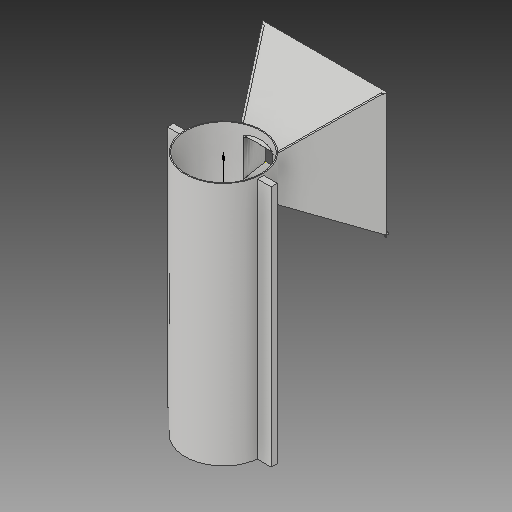
# Autodesk Inventor part: cilindro exterior
Saved by Autodesk Inventor 2019 (Build 230136000, 136)
## iProperties
Created: 2021-07-01
Part Number: cilindro exterior
Material: Genérico
Document SubType Name: Modeling
Designer: Usuario
Density: 1 g/cm^3
Appearance: Valor por defecto
Author: Usuario
Autodesk Inventor part; units mm, degrees
ref_plane "XZ Plane" through (0, 0, 0) normal (0, 1, 0) x (-1, 0, 0)
sketch "Boceto1" plane through (0, 0, 0) normal (0, 0, 1) x (1, 0, 0)
  line L0 (0, 0) -> (0, 625)
  line L1 (0, 625) -> (35, 625)
  line L2 (35, 625) -> (35, 0)
  line L3 (35, 0) -> (0, 0)
  dimension "d0" = 625
  dimension "d1" = 35
  constraints: 8 end point, 3 perpendicular, 1 vertical
  measures "d0" distance of L0.start L0.end
  measures "d1" distance of L0.end L1.end
extrude "Extrusión1" add sketch "Boceto1" along normal blind 5
sketch "Boceto2" plane through (0, 0, 0) normal (0, -1, 0) x (1, 0, 0)
  line L0 (0, 5) -> (35, 5) projected
  line L1 (35, 5) -> (133.75, 5)
  circle A0 centre (133.75, 5) radius 98.75
  line L2 (133.75, 5) -> (267.5, 5)
  line L3 (267.5, 5) -> (267.5, 0)
  line L4 (267.5, 0) -> (232.5, 0)
  line L5 (232.5, 0) -> (232.5, 5)
  circle A1 centre (133.75, 5) radius 96.25
  point P0 (0, 0)
  dimension "d5" = 197.5
  dimension "d4" = 98.75
  dimension "d6" = 133.75
  dimension "d7" = 5
  dimension "d8" = 35
  dimension "d14" = 192.5
  constraints: 10 end point, 2 coincident, 2 horizontal, 2 perpendicular, 1 centre point, 1 horizontal alignment, 1 point on line, 2 other
  measures "d4" distance of L0.end L1.end
  measures "d6" distance of L2.start L2.end
  measures "d7" distance of L2.end L3.end
  measures "d8" distance of L3.end L4.end
  measures "d14" diameter of A1
extrude "Extrusión2" add sketch "Boceto2" against normal blind 625
sketch "Boceto3" plane through (0, 0, 0) normal (0, -1, 0) x (1, 0, 0)
  arc A0 (35, 5) -> (232.5, 5) centre (133.75, 5) ccw projected
  line L0 (133.75, 5) -> (133.75, -93.75)
  circle A1 centre (133.75, 5) radius 12.5
  point P0 (0, 0)
  dimension "d11" = 25
  constraints: 2 end point, 1 centre point, 1 coincident, 1 point on circle, 1 vertical
  measures "d11" diameter of A1
extrude "Extrusión3" cut sketch "Boceto3" against normal blind 625
sketch "Boceto4" plane through (0, 625, 0) normal (0, 1, 0) x (1, 0, 0)
  circle A0 centre (133.75, -5) radius 12.5 projected
  circle A1 centre (133.75, -5) radius 96.25
  point P0 (0, 0)
  dimension "d15" = 192.5
  constraints: 1 centre point, 1 coincident
  measures "d15" diameter of A1
extrude "Extrusión4" cut sketch "Boceto4" against normal blind 620
ref_plane "Plano de trabajo1" through (133.75, 0, -93.75) normal (0, 0, 1) x (1, 0, 0)
sketch "Boceto5" plane through (133.75, 0, -93.75) normal (0, 0, 1) x (1, 0, 0)
  line L0 (98.75, 625) -> (-98.75, 625) projected
  line L1 (0, 625) -> (0, 600)
  line L2 (0, 600) -> (55, 600)
  line L3 (55, 600) -> (55, 550)
  line L4 (55, 550) -> (55, 500)
  line L5 (55, 500) -> (0, 500)
  line L6 (0, 500) -> (-55, 500)
  line L7 (-55, 500) -> (-55, 600)
  line L8 (-55, 600) -> (0, 600)
  point P0 (-133.75, 0)
  dimension "d18" = 25
  dimension "d19" = 55
  dimension "d20" = 50
  dimension "d21" = 50
  dimension "d22" = 55
  constraints: 16 end point, 5 perpendicular, 4 point on line, 1 midpoint, 1 vertical
  measures "d18" distance of L1.start L1.end
  measures "d19" distance of L1.end L2.end
  measures "d20" distance of L2.end L3.end
  measures "d21" distance of L3.end L4.end
  measures "d22" distance of L5.end L6.end
extrude "Extrusión5" cut sketch "Boceto5" along normal blind 10
ref_plane "Plano de trabajo2" through (133.75, 0, 0) normal (1, 0, 0) x (0, 1, 0)
sketch "Boceto6" plane through (133.75, 0, 0) normal (1, 0, 0) x (0, 1, 0)
  line L0 (500, -83.75) -> (600, -83.75)
  line L1 (500, -258.75) -> (218.701741, -265.847227)
  line L2 (500, -258.75) -> (941.5108, -258.75)
  line L3 (500, -83.75) -> (450.417, -169.630275)
  line L4 (500, -83.75) -> (599.166, -83.75) construction
  line L5 (450.417, -169.630275) -> (397.470182, -261.336854)
  line L6 (599.166, -83.75) -> (812.26, -83.75) construction
  line L7 (708.977475, -258.75) -> (599.166, -83.75)
  line L8 (392.471773, -261.462965) -> (495.771773, -82.542116)
  line L9 (714.880332, -258.75) -> (605.068857, -83.75)
  line L10 (500, -258.75) -> (394.038104, -258.75)
  line L11 (399.996368, -256.961371) -> (707.855121, -256.961371)
  line L12 (605.068857, -83.75) -> (600.83362, -86.407587)
  line L13 (493.540042, -86.407587) -> (497.234242, -88.540434)
  point P0 (0, 0)
  dimension "d25" = 175
  dimension "d26" = 99.166
  dimension "d27" = 120
  dimension "d30" = 206.6
  dimension "d31" = 5
  dimension "d32" = 206.6
  dimension "d33" = 5
  dimension "d34" = 1.78863
  constraints: 26 end point, 13 point on line, 3 horizontal, 3 parallel, 2 perpendicular, 1 equal length
  measures "d25" distance of L0.start L1.start
  measures "d26" distance of L0.start L3.end
  measures "d27" angle of L3 L4
  measures "d30" distance of L8.start L8.end
  measures "d31" distance of L5.end L8.start
  measures "d32" distance of L9.start L9.end
  measures "d33" distance between parallel lines of L7 L9
  measures "d34" distance between parallel lines of L11 L2
extrude "Extrusión6" add sketch "Boceto6" along normal mid plane 98 contours L3 L5 L10 L8 L13 | L12 L9 L2 L7 | L10 L5 L1 L8
sketch "Boceto9" plane through (84.75, 708.977475, -258.75) normal (0, -0.8470474, -0.5315173) x (1, 0, 0)
  line L0 (86.365969, 203.462529) -> (98, 203.462529)
  line L1 (98, 203.462529) -> (98, 0)
  line L2 (98, 203.462529) -> (98, 0)
  line L3 (98, 0) -> (0, 0)
  line L4 (98, 0) -> (0, 0)
  line L5 (98, 0) -> (209, 0)
  line L6 (0, 0) -> (-111, 0)
  line L7 (-111, 0) -> (0, 203.462529)
  line L8 (98, 203.462529) -> (209, 0)
  line L9 (0, 0) -> (0, 203.462529)
  line L10 (0, 0) -> (0, 203.462529)
  point P0 (-84.75, 596.007319)
  dimension "d40" = 111
  dimension "d41" = 111
  constraints: 14 end point, 2 collinear, 2 horizontal, 1 vertical
  measures "d40" distance of L1.end L5.end
  measures "d41" distance of L3.end L6.end
extrude "Extrusión8" add sketch "Boceto9" against normal blind 5
sketch "Boceto10" plane through (84.75, 0, 0) normal (-1, 0, 0) x (0, 0, 1)
  line L0 (-256.092413, 713.212712) -> (-258.75, 714.880332)
  line L1 (-256.092413, 713.212712) -> (-258.75, 714.880332)
  line L2 (-258.75, 714.880332) -> (-258.75, 708.977475)
  line L3 (-258.75, 708.977475) -> (-256.092413, 713.212712)
  line L4 (-258.75, 714.880332) -> (-258.75, 708.977475)
  line L5 (-258.75, 708.977475) -> (-256.092413, 713.212712)
  point P0 (0, 0)
  constraints: 7 end point, 1 collinear, 1 vertical
extrude "Extrusión9" cut sketch "Boceto10" against normal blind 300
sketch "Boceto11" plane through (84.75, 397.470182, -261.336854) normal (0, 0.8660254, -0.5) x (1, 0, 0)
  line L0 (0, 0) -> (98, 0)
  line L1 (0, 0) -> (98, 0)
  line L2 (98, 0) -> (209, 0)
  line L3 (98, 0) -> (98, -199.528119)
  line L4 (98, 0) -> (98, -199.528119)
  line L5 (98, -199.528119) -> (209, 0)
  line L6 (0, 0) -> (-111, 0)
  line L7 (0, -199.528119) -> (0, 0)
  line L8 (-111, 0) -> (0, -199.528119)
  line L9 (0, -199.528119) -> (0, 0)
  point P0 (-84.75, -27.589263)
  dimension "d46" = 98
  dimension "d47" = 111
  dimension "d48" = 111
  constraints: 14 end point, 2 horizontal, 1 collinear, 1 perpendicular, 1 point on line
  measures "d46" distance of L0.start L0.end
  measures "d47" distance of L0.end L2.end
  measures "d48" distance of L0.start L6.end
extrude "Extrusión10" add sketch "Boceto11" against normal blind 4.27
sketch "Boceto12" plane through (182.75, 0, 0) normal (1, 0, 0) x (0, 0, -1)
  line L0 (261.336854, 397.470182) -> (88.540434, 497.234242)
  line L1 (261.336854, 397.470182) -> (259.204007, 393.775983)
  line L2 (259.204007, 393.775983) -> (261.462965, 392.471773)
  line L3 (259.204007, 393.775983) -> (261.462965, 392.471773)
  line L4 (261.462965, 392.471773) -> (261.336854, 397.470182)
  line L5 (261.462965, 392.471773) -> (261.336854, 397.470182)
  point P0 (0, 0)
  constraints: 6 end point, 2 collinear, 1 perpendicular
extrude "Extrusión11" cut sketch "Boceto12" against normal blind 3000
ref_plane "Plano de trabajo6" through (0, 550, 0) normal (0, 1, 0) x (1, 0, 0)
sketch "Boceto19" plane through (0, 550, 0) normal (0, 1, 0) x (1, 0, 0)
  line L0 (-26.25, 256.092413) -> (84.75, 83.75)
  line L1 (84.75, 86.407587) -> (84.75, 83.75)
  line L2 (-26.25, 256.092413) -> (84.75, 83.75)
  line L3 (84.75, 83.75) -> (86.176529, 81.535122)
  arc A0 (232.5, -5) -> (35, -5) centre (133.75, -5) ccw
  line L4 (86.176529, 81.535122) -> (181.323471, 81.535122)
  line L5 (182.75, 83.75) -> (293.75, 256.092413)
  line L6 (181.323471, 81.535122) -> (293.75, 256.092413)
  line L7 (293.75, 256.092413) -> (-26.25, 256.092413)
  line L8 (293.75, 256.092413) -> (-26.25, 256.092413)
  line L9 (-26.25, 256.092413) -> (293.75, 256.092413)
  line L10 (92.123843, 81.535122) -> (-17.082353, 251.092413)
  line L11 (-17.082353, 251.092413) -> (284.582353, 251.092413)
  line L12 (90.44873, 83.75) -> (177.05127, 83.75)
  line L13 (86.176529, 81.535122) -> (181.323471, 81.535122)
  line L14 (182.75, 83.75) -> (90.44873, 83.75)
  line L15 (96.500839, 83.75) -> (170.999161, 83.75)
  line L16 (90.44873, 83.75) -> (-20.302686, 256.092413)
  line L17 (-26.25, 256.092413) -> (-20.302686, 256.092413)
  line L18 (287.795258, 256.092413) -> (289.502973, 258.75)
  line L19 (293.75, 258.75) -> (-26.25, 258.75)
  line L20 (171.115969, 86.407587) -> (182.75, 86.407587)
  line L21 (287.802686, 256.092413) -> (293.75, 256.092413)
  line L22 (165.400429, 88.540434) -> (182.75, 88.540434)
  line L23 (180.129511, 88.540434) -> (177.05127, 83.75)
  line L24 (284.582353, 251.092413) -> (177.05127, 83.75)
  line L25 (177.05127, 83.75) -> (284.582353, 251.092413)
  line L26 (284.582353, 251.092413) -> (287.795258, 256.092413)
  point P0 (0, 0)
  dimension "d61" = 5
  dimension "d63" = 5
  constraints: 38 end point, 8 point on line, 6 collinear, 5 horizontal, 4 point on circle
  measures "d61" distance between parallel lines of L0 L10
  measures "d63" distance between parallel lines of L7 L11
extrude "Extrusión12" add sketch "Boceto19" along normal mid plane 320 contours L7 L16 A0 L3 L0 | L7 L5 L14 L23 L24 L26 | A0 L14 L6
sketch "Boceto20" plane through (287.795258, 400.498061, -256.092413) normal (-0.8412841, 0, -0.5405933) x (-0.5405933, 0, 0.8412841)
  line L0 (0, 0) -> (0, 307.253704)
  line L1 (205.829184, 200.335559) -> (201.69742, 200.335559)
  line L2 (0, 307.253704) -> (201.69742, 200.335559)
  line L3 (205.829184, 93.041981) -> (201.69742, 93.041981)
  line L4 (201.69742, 200.335559) -> (201.69742, 93.041981)
  line L5 (0, -4.930571) -> (194.314764, 89.451138)
  line L6 (201.69742, 93.041981) -> (0, -4.930571)
  line L7 (0, -10.498061) -> (0, -4.930571)
  line L8 (0, -4.930571) -> (0, -10.498061)
  line L9 (204.856385, -10.498061) -> (0, -10.498061)
  line L10 (0, -10.498061) -> (204.856385, -10.498061)
  line L11 (204.856385, -10.498061) -> (205.829184, 93.041981)
  line L12 (2.870843, 309.501939) -> (-2.715479, 309.501939)
  line L13 (204.410203, 309.501939) -> (2.870843, 309.501939)
  line L14 (2.870843, 309.501939) -> (204.410203, 309.501939)
  line L15 (204.856385, 204.570796) -> (6.085825, 309.501939)
  line L16 (204.410203, 309.501939) -> (204.856385, 204.570796)
  line L17 (204.856385, 204.570796) -> (6.085825, 309.501939)
  point P0 (371.026655, -400.498061)
  constraints: 20 end point, 2 vertical, 1 collinear, 1 horizontal, 1 parallel, 1 perpendicular
extrude "Extrusión13" cut sketch "Boceto20" against normal blind 320
sketch "Boceto31" plane through (-20.302686, 400.498061, -256.092413) normal (0.8412676, 0, -0.540619) x (-0.540619, 0, -0.8412676)
  line L0 (-204.414072, -10.498061) -> (3.215231, -10.498061)
  line L1 (-204.8604, -10.498061) -> (-204.8604, 99.501939)
  line L2 (7.627208, -3.027879) -> (-165.370858, -3.027879)
  line L3 (2.135385, -4.930571) -> (5.831102, -6.725807)
  line L4 (7.627208, -3.027879) -> (5.831102, -6.725807)
  line L5 (0, -10.498061) -> (-204.8604, -10.498061)
  line L6 (0, -10.498061) -> (-204.414072, -10.498061)
  line L7 (-204.8604, 99.501939) -> (-208.132285, 99.501939)
  line L8 (-204.414072, -10.498061) -> (-204.8604, 99.501939)
  line L9 (-194.319279, 89.451481) -> (0, -4.930571)
  line L10 (-204.8604, 99.501939) -> (0, -4.930571)
  line L11 (0, -4.930571) -> (0, -10.498061)
  point P0 (-226.418262, -400.498061)
  constraints: 10 end point, 1 collinear
extrude "Extrusión21" cut sketch "Boceto31" against normal blind 175 contours L8 L10 L2 L9 L11 L0 | L9 L2 L10
sketch "Boceto32" plane through (90.44873, 625, -83.75) normal (0.8412676, 0, -0.540619) x (-0.540619, 0, -0.8412676)
  line L0 (0.446328, 0) -> (0.446328, 85)
  line L1 (201.985694, 85) -> (0.446328, 85)
  line L2 (0.446328, 85) -> (201.985694, 85)
  line L3 (0, -25) -> (0, -19.931143)
  line L4 (201.985694, 85) -> (0, -19.931143)
  line L5 (0, 0) -> (0, 85)
  line L6 (0, 85) -> (0, -19.931143)
  line L7 (0, 85) -> (1.071476, 85)
  point P0 (-21.557862, -625)
  constraints: 8 end point, 1 horizontal, 1 point on line
extrude "Extrusión22" cut sketch "Boceto32" against normal blind 175
sketch "Boceto33" plane through (177.05127, 605.068857, -83.75) normal (0.5405884, -0.0042521, -0.8412765) x (-0.8412841, 0, -0.5405933)
  line L0 (-4.791483, 104.932091) -> (0, 104.932091)
  line L1 (-4.791483, 104.932091) -> (0, 104.932091)
  line L2 (0, 19.930963) -> (0, 104.930194)
  line L3 (0, 104.932091) -> (0, 19.930963)
  ellipse E0 centre (-11.548986, 19.513949) end of major axis (-110.298986, 19.513949) minor radius 0.419895 (0, 19.930963) -> (-0.743957, 19.931323) ccw
  line L4 (0, 19.930963) -> (0, 19.930963)
  line L5 (0, 19.930963) -> (0, 19.930963)
  line L6 (-0.743957, 19.931323) -> (-4.791483, 104.932091)
  line L7 (0, 19.930963) -> (0, 0)
  line L8 (-0.743957, 19.931323) -> (0, 19.930963)
  point P0 (103.675725, -605.76996)
  constraints: 12 end point, 2 collinear, 2 perpendicular, 1 other
extrude "Extrusión23" cut sketch "Boceto33" against normal blind 10
sketch "Boceto35" plane through (90.207437, 390, -84.125481) normal (-0.5406145, 0.0040575, -0.8412607) x (-0.8412676, 0, 0.540619)
  ellipse E0 centre (11.551977, 0.399737) end of major axis (-87.198023, 0.399737) minor radius 0.400677 (0, 0.001811) -> (4.791469, 0) ccw
  line L0 (0, 0.001811) -> (4.791469, 0)
  line L1 (0, 0.001811) -> (0, 215.068898)
  line L2 (4.791469, 0) -> (0, 110.000905)
  line L3 (0, 110.000905) -> (0, 0.001811)
  line L4 (0, 0.001811) -> (4.791469, 0)
  point P0 (121.368422, -389.907508)
  constraints: 8 end point, 1 collinear, 1 other
extrude "Extrusión25" cut sketch "Boceto35" against normal blind 10
sketch "Boceto36" plane through (133.75, 5, 5) normal (0, 1, 0) x (1, 0, 0)
  circle A0 centre (0, 0) radius 96.25
  circle A1 centre (0, 0) radius 98.75
  point P0 (-133.75, 5)
  constraints: 2 centre point, 1 coincident
extrude "Extrusión26" add sketch "Boceto36" along normal blind 625
sketch "Boceto37" plane through (133.75, 0, -93.75) normal (0, 0, 1) x (1, 0, 0)
  line L0 (43.30127, 605.068857) -> (43.30127, 493.540042)
  line L1 (43.30127, 600.98534) -> (0, 605.440941)
  ellipse E0 centre (0, 543.475895) end of major axis (-98.75, 543.475895) minor radius 61.965047 (37.365969, 600.83362) -> (-37.365969, 600.83362) ccw
  ellipse E1 centre (0, 543.475895) end of major axis (-96.25, 543.475895) minor radius 60.396311 (30.14491, 600.83362) -> (-30.14491, 600.83362) ccw
  line L2 (0, 603.872206) -> (-43.30127, 600.83362)
  line L3 (-45.0091, 600.83362) -> (-37.365969, 600.83362)
  line L4 (-43.30127, 500) -> (-43.30127, 605.068857)
  line L5 (-43.30127, 600.83362) -> (-43.30127, 500)
  line L6 (-43.30127, 500) -> (0, 494.226497)
  ellipse E2 centre (0, 551.239836) end of major axis (98.75, 551.239836) minor radius 57.013339 (-31.650429, 497.234242) -> (31.650429, 497.234242) ccw
  line L7 (43.30127, 497.234242) -> (43.30127, 600.98534)
  line L8 (43.30127, 497.234242) -> (31.650429, 497.234242)
  line L9 (31.650429, 497.234242) -> (0, 494.226497)
  point P0 (-133.75, 0)
  constraints: 14 end point, 2 point on line, 1 collinear, 1 horizontal, 1 parallel, 6 other
extrude "Extrusión27" cut sketch "Boceto37" along normal blind 10 contours L0 L8 L9 L6 L4 L3 E0 L1 | L2 E1
sketch "Boceto38" plane through (-26.25, 393.772254, -259.201854) normal (-0.8738763, 0.2430742, 0.4210168) x (0.4861484, 0.4369381, 0.7567991)
  line L0 (4.108673, 0) -> (0, 0)
  line L1 (0, 4.27) -> (0, 0)
  line L2 (0, 0) -> (0, 4.27)
  line L3 (0, 4.27) -> (5.296918, 4.27)
  line L4 (0, 4.27) -> (6.929766, 4.27)
  line L5 (3.137629, 0) -> (0, 0)
  line L6 (3.137629, 0) -> (5.296918, 4.27)
  constraints: 8 end point, 1 perpendicular, 1 point on line, 1 vertical
sketch "Boceto40" plane through (232.5, 0, 5) normal (0, 0, 1) x (1, 0, 0)
  line L0 (0, 625) -> (35, 625) projected
  line L1 (0, 625) -> (35, 625)
  line L2 (0, 0) -> (35, 0) projected
  line L3 (35, 625) -> (35, 0)
  line L4 (35, 0) -> (0, 0)
  line L5 (0, 0) -> (0, 625) projected
  line L6 (0, 0) -> (0, 625)
  point P0 (-232.5, 0)
  constraints: 8 end point, 2 perpendicular, 1 collinear, 1 horizontal
extrude "Extrusión28" add sketch "Boceto40" along normal blind 11
sketch "Boceto41" plane through (0, 0, 5) normal (0, 0, 1) x (1, 0, 0)
  line L0 (0, 625) -> (0, 0) projected
  line L1 (35, 0) -> (35, 625) projected
  line L2 (0, 625) -> (35, 625)
  line L3 (35, 625) -> (35, 0)
  line L4 (0, 0) -> (35, 0) projected
  line L5 (35, 0) -> (0, 0)
  line L6 (0, 0) -> (0, 625)
  constraints: 8 end point, 2 perpendicular, 1 collinear, 1 horizontal
extrude "Extrusión29" add sketch "Boceto41" along normal blind 11
ref_plane "Plano de trabajo10" through (232.5, 0, 0) normal (1, 0, 0) x (0, 1, 0)
sketch "Boceto42" plane through (232.5, 0, 0) normal (1, 0, 0) x (0, 1, 0)
  line L0 (0, 0) -> (50, 0)
  line L1 (0, 0) -> (625, 0) projected
  line L2 (50, 0) -> (50, -20)
  line L3 (50, -20) -> (100, -20)
  line L4 (100, -20) -> (100, -60)
  line L5 (100, -60) -> (50, -60)
  line L6 (50, -60) -> (50, -20)
  dimension "d105" = 50
  dimension "d106" = 20
  dimension "d107" = 50
  dimension "d108" = 40
  constraints: 12 end point, 4 perpendicular, 2 point on line, 1 vertical
  measures "d105" distance of L0.start L0.end
  measures "d106" distance of L0.end L2.end
  measures "d107" distance of L2.end L3.end
  measures "d108" distance of L3.end L4.end
extrude "Extrusión30" cut sketch "Boceto42" against normal blind 20
ref_plane "Plano de trabajo11" through (35, 0, 0) normal (1, 0, 0) x (0, 1, 0)
sketch "Boceto44" plane through (35, 0, 0) normal (1, 0, 0) x (0, 1, 0)
  line L0 (0, 0) -> (0, 16) projected
  line L1 (0, 0) -> (630, 0)
  line L2 (630, 101.25) -> (630, -91.25) projected
  line L3 (0, 0) -> (625, 0) projected
  line L4 (312.5, 0) -> (312.5, 35)
  line L5 (312.5, 35) -> (312.5, 50)
  line L6 (312.5, 50) -> (354.5, 50)
  line L7 (354.5, 50) -> (354.5, 80)
  line L8 (354.5, 80) -> (254.5, 80)
  line L9 (254.5, 80) -> (254.5, 50)
  line L10 (254.5, 50) -> (312.5, 50)
  dimension "d116" = 35
  dimension "d117" = 15
  dimension "d118" = 42
  dimension "d119" = 30
  dimension "d120" = 100
  constraints: 16 end point, 5 perpendicular, 3 point on line, 1 horizontal, 1 midpoint, 1 vertical
  measures "d116" distance of L4.start L4.end
  measures "d117" distance of L4.end L5.end
  measures "d118" distance of L5.end L6.end
  measures "d119" distance of L6.end L7.end
  measures "d120" distance of L7.end L8.end
extrude "Extrusión31" cut sketch "Boceto44" along normal blind 50
